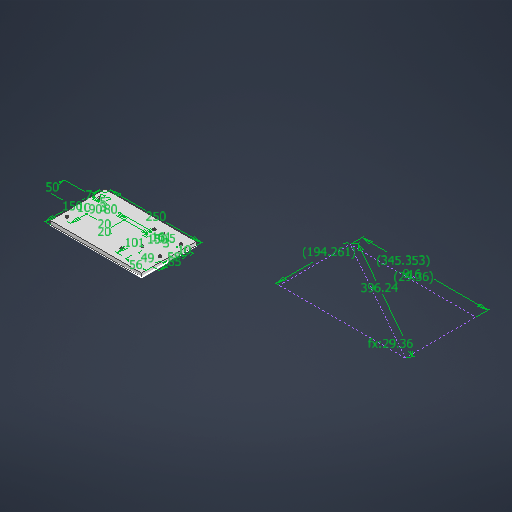
# Autodesk Inventor part: Main Mount
Saved by Autodesk Inventor 2025.1 (Build 291241000, 241)
## iProperties
Created: 2025-02-09
Part Number: Main Mount
Material: Generic
Document SubType Name: Modeling
Designer: jerem
Density: 1 g/cm^3
Appearance: Default
Author: jerem
Autodesk Inventor part; units mm, degrees
ref_plane "YZ Plane" through (0, 0, 0) normal (1, 0, 0) x (0, 1, 0)
ref_plane "XZ Plane" through (0, 0, 0) normal (0, 1, 0) x (-1, 0, 0)
ref_plane "XY Plane" through (0, 0, 0) normal (0, 0, 1) x (1, 0, 0)
sketch "Sketch1" plane through (0, 0, 0) normal (0, 1, 0) x (-1, 0, 0)
  line L0 (-333.2556, -289.2611) -> (-678.6087, -289.2611) construction
  line L1 (-678.6087, -289.2611) -> (-678.6087, -95) construction
  line L2 (-678.6087, -95) -> (-333.2556, -95) construction
  line L3 (-333.2556, -95) -> (-333.2556, -289.2611) construction
  line L4 (-333.2556, -289.2611) -> (-678.6087, -95) construction
  line L5 (-488.8826, -290.1866) -> (-488.8826, -299.1866) construction
  line L6 (-488.8826, -299.1866) -> (-504.8826, -299.1866) construction
  line L7 (-488.8826, -290.1866) -> (-504.8826, -299.1866) construction
  line L8 (45, -10.5) -> (45, 9.5)
  line L9 (110, 44.5) -> (110, -45.5) construction
  circle A0 centre (110, 44.5) radius 1.5
  line L10 (115, -50.5) -> (115, 50.5) construction
  line L11 (110, -45.5) -> (-40, -45.5) construction
  line L12 (-46, -50.5) -> (115, -50.5) construction
  line L13 (115, 50.5) -> (-46, 50.5) construction
  line L14 (-40, 44.5) -> (110, 44.5) construction
  line L15 (25, -10.5) -> (45, -10.5)
  line L16 (25, 9.5) -> (25, -10.5)
  line L17 (25, -10.5) -> (45, 9.5) construction
  line L18 (45, -10.5) -> (25, 9.5) construction
  line L19 (45, 9.5) -> (25, 9.5)
  line L20 (-46, 50.5) -> (-46, -50.5) construction
  line L21 (-40, -45.5) -> (-40, 44.5) construction
  circle A1 centre (-40, 44.5) radius 1.5
  circle A2 centre (-40, -45.5) radius 1.5
  circle A3 centre (110, -45.5) radius 1.5
  line L22 (110, -45.5) -> (110, -50.5) construction
  line L23 (110, -45.5) -> (115, -45.5) construction
  line L24 (-59, -50.5) -> (-115, -50.5) construction
  line L25 (-115, -50.5) -> (-115, 34.5) construction
  line L26 (-115, 34.5) -> (-59, 34.5) construction
  line L27 (-59, 34.5) -> (-59, -50.5) construction
  line L28 (-62.5, -47) -> (-111.5, -47) construction
  line L29 (-111.5, -47) -> (-111.5, 11) construction
  line L30 (-111.5, 11) -> (-62.5, 11) construction
  line L31 (-62.5, 11) -> (-62.5, -47) construction
  circle A4 centre (-62.5, -47) radius 1.5
  circle A5 centre (-111.5, -47) radius 1.5
  circle A6 centre (-62.5, 11) radius 1.5
  circle A7 centre (-111.5, 11) radius 1.5
  line L32 (-87, -47) -> (-87, -50.5) construction
  line L33 (-125, 75) -> (125, 75)
  line L34 (125, 75) -> (125, -75)
  line L35 (125, -75) -> (-125, -75)
  line L36 (-125, -75) -> (-125, 75)
  line L37 (-125, 75) -> (125, -75) construction
  line L38 (125, 75) -> (-125, -75) construction
  line L39 (0, -57.5) -> (0, -75)
  line L40 (115, 0) -> (125, 0) construction
  circle A8 centre (110, -45.5) radius 3.5
  circle A9 centre (110, 44.5) radius 3.5
  circle A10 centre (-40, 44.5) radius 3.5
  circle A11 centre (-40, -45.5) radius 3.5
  circle A12 centre (-62.5, -47) radius 3.5
  circle A13 centre (-62.5, 11) radius 3.5
  circle A14 centre (-111.5, 11) radius 3.5
  circle A15 centre (-111.5, -47) radius 3.5
  point P0 (0, 0)
  point P1 (35, -0.5)
  dimension "d34" = 396.24
  dimension "d37" = 345.3531
  dimension "d39" = 9
  dimension "d40" = 16
  dimension "d41" = 29.358
  dimension "d42" = 29.358
  dimension "d43" = 194.2611
  dimension "d46" = 161
  dimension "d47" = 101
  dimension "d48" = 3
  dimension "d49" = 150
  dimension "d50" = 90
  dimension "d51" = 5
  dimension "d52" = 20
  dimension "d53" = 20
  dimension "d54" = 50
  dimension "d55" = 80
  dimension "d56" = 56
  dimension "d57" = 85
  dimension "d58" = 49
  dimension "d59" = 58
  dimension "d60" = 3
  dimension "d61" = 3.5
  dimension "d64" = 250
  dimension "d65" = 150
  dimension "d73" = 10
  dimension "d74" = 10
  dimension "d75" = 7
  constraints: 82 end point, 16 centre point, 15 coincident, 14 parallel, 12 equal radius, 11 perpendicular, 9 midpoint, 8 horizontal, 3 point on line, 2 vertical, 1 collinear, 1 tangent
  measures "d34" distance of L0.start L1.end
  measures "d37" distance of L0.start L0.end
  measures "d39" distance of L5.start L5.end
  measures "d40" distance of L5.end L6.end
  measures "d41" angle of L6 L7
  measures "d42" angle of L2 L4
  measures "d43" distance of L2.end L0.start
  measures "d46" distance of L12.end L12.start
  measures "d47" distance of L12.start L13.end
  measures "d48" diameter of A3
  measures "d49" distance of L11.start L11.end
  measures "d50" distance of L14.end L11.start
  measures "d51" distance of L11.start L22.end
  measures "d52" distance of L16.start L17.end
  measures "d53" distance of L17.end L15.end
  measures "d54" distance from line of L12 point (35, -0.5)
  measures "d55" distance from line of L10 point (35, -0.5)
  measures "d56" distance of L26.start L27.start
  measures "d57" distance of L24.end L26.start
  measures "d58" distance of L30.start L31.start
  measures "d59" distance of L28.end L30.start
  measures "d60" diameter of A4
  measures "d61" distance between parallel lines of L24 L28
  measures "d64" distance of L34.end L35.end
  measures "d65" distance of L33.end L34.end
  measures "d73" distance between parallel lines of L34 L10
  measures "d74" distance between parallel lines of L36 L25
  measures "d75" diameter of A8
extrude "Extrusion2" add sketch "Sketch1" along normal blind 10 contours L15 L16 L19 L8 | A0 | A1 | A2 | A3 | A4 | A5 | A6 | A7 | L33 L34 L35 L36 | A8 | A9 | A10 | A11 | A12 | A13 | A14 | A15
extrude "Extrusion3" add sketch "Sketch1" along normal blind 2 from surface at 10 contours A8 | A9 | A10 | A11 | A12 | A13 | A14 | A15
body "Solid2"
